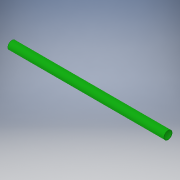
# Autodesk Inventor part: Bottom Roller
Saved by Autodesk Inventor 2017 (Build 210142000, 142)
## iProperties
Created: 2017-01-14
Part Number: Bottom Roller
Material: Generic
Document SubType Name: Modeling
Designer: Ben
Density: 1 g/cm^3
Appearance: Dark Green
Author: Ben
Autodesk Inventor part; units mm, degrees
ref_plane "YZ Plane" through (0, 0, 0) normal (1, 0, 0) x (0, 1, 0)
ref_plane "XZ Plane" through (0, 0, 0) normal (0, 1, 0) x (-1, 0, 0)
ref_plane "XY Plane" through (0, 0, 0) normal (0, 0, 1) x (1, 0, 0)
sketch "Sketch1" plane through (0, 0, 0) normal (1, 0, 0) x (0, 1, 0)
  circle A0 centre (0, 0) radius 15.875
  circle A1 centre (0, 0) radius 14.6304
  dimension "d0" = 31.75
  dimension "d4" = 1.2446
  constraints: 2 centre point, 2 coincident
  measures "d0" diameter of A0
  measures "d4" radial gap between concentric circles of A0 A1
extrude "Extrusion1" add sketch "Sketch1" along normal mid plane 596.9
body "Solid1"
